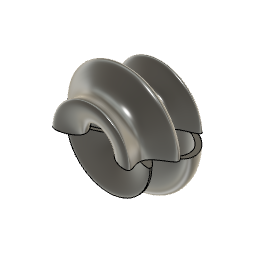
Abstract Circle v1 (Autodesk Fusion 360 design; units mm, degrees)
Autodesk Fusion 360 part; units mm, degrees
sketch "Sketch1" plane through (0, 0, 0) normal (0, 0, 1) x (1, 0, 0)
  spline S0 degree 5 poles (0, 0) (-1.4662, 0.7183) (-4.2888, 2.1966) (-8.0702, 4.4991) (-11.7581, 7.5956) (-13.3358, 11.2313) (-11.5888, 14.4429) (-6.8157, 17.1384) (-0.0929, 19.3357) (6.9956, 21.1422) (12.7502, 22.7235) (15.7261, 24.2765) (15.0691, 26.0007) (10.9795, 28.0708) (4.6166, 30.6078) (-2.3647, 33.6525) (-8.1726, 37.1355) (-11.2612, 40.8524) (-10.7466, 44.4259) (-6.6786, 47.3053) (0.2549, 48.9047) (8.9284, 48.7162) (18.0189, 46.4407) (26.218, 42.0947) (32.4803, 36.1725) (36.0989, 29.5147) (36.7231, 23.082) (34.4003, 17.7561) (29.601, 14.139) (23.273, 12.3295) (16.8297, 11.7745) (11.7686, 11.5977) (9.3075, 10.8895) (10.061, 8.9801) (13.5787, 5.7975) (18.5062, 1.8253) (23.1284, -2.1837) (25.7913, -5.4169) (25.3793, -7.2462) (21.7551, -7.4496) (15.5084, -6.1106) (9.277, -4.0415) (4.5082, -2.1134) (1.4662, -0.7183) (0, 0) knots 0 0 0 0 0 0 0.025 0.05 0.075 0.1 0.125 0.15 0.175 0.2 0.225 0.25 0.275 0.3 0.325 0.35 0.375 0.4 0.425 0.45 0.475 0.5 0.525 0.55 0.575 0.6 0.625 0.65 0.675 0.7 0.725 0.75 0.775 0.8 0.825 0.85 0.875 0.9 0.925 0.95 0.975 1 1 1 1 1 1
  spline S1 degree 5 poles (25, -5) (25.2012, -4.493) (25.9112, -3.5734) (27.8624, -2.4724) (31.8799, -1.4172) (37.7823, -0.0737) (42.9674, 2.0791) (46.1535, 5.639) (46.8953, 10.7059) (45.8562, 16.7195) (44.277, 22.7729) (43.572, 27.8507) (44.9021, 31.0817) (48.7004, 32.018) (54.3847, 30.8082) (60.8161, 27.9506) (66.6355, 24.1148) (70.6443, 19.939) (72.1699, 15.8366) (71.4326, 11.8025) (69.1917, 7.6017) (66.3861, 2.9629) (63.815, -2.2522) (61.7159, -7.8168) (59.6962, -13.1205) (57.1028, -17.417) (53.2953, -20.013) (47.9246, -20.4592) (41.2901, -18.7958) (34.3829, -15.5854) (28.4685, -11.6354) (25.5217, -8.5658) (24.7041, -6.6154) (24.7988, -5.507) (25, -5) knots 0 0 0 0 0 0 0.033333 0.066667 0.1 0.133333 0.166667 0.2 0.233333 0.266667 0.3 0.333333 0.366667 0.4 0.433333 0.466667 0.5 0.533333 0.566667 0.6 0.633333 0.666667 0.7 0.733333 0.766667 0.8 0.833333 0.866667 0.9 0.933333 0.966667 1 1 1 1 1 1
  spline S2 degree 5 poles (35, -10) (35.0607, -10.4295) (35.3776, -11.294) (36.4362, -12.596) (38.8816, -14.2347) (42.9641, -15.6792) (47.2397, -16.0554) (50.9557, -15.0177) (53.6877, -12.5043) (55.4948, -8.8331) (56.7094, -4.5257) (57.7882, -0.1787) (59.1317, 3.6928) (60.9403, 6.7779) (62.9942, 9.1614) (64.7162, 11.2631) (65.4865, 13.5525) (64.8535, 16.3559) (62.8604, 19.5601) (60.044, 22.6144) (57.1287, 24.8092) (54.8042, 25.4812) (53.4723, 24.2451) (52.9956, 21.2235) (52.8887, 16.8909) (52.5156, 11.9109) (51.2934, 6.9702) (48.87, 2.632) (45.3722, -0.8609) (41.3906, -3.5951) (37.7274, -5.8274) (35.7154, -7.4638) (35.0136, -8.7169) (34.9393, -9.5705) (35, -10) knots 0 0 0 0 0 0 0.033333 0.066667 0.1 0.133333 0.166667 0.2 0.233333 0.266667 0.3 0.333333 0.366667 0.4 0.433333 0.466667 0.5 0.533333 0.566667 0.6 0.633333 0.666667 0.7 0.733333 0.766667 0.8 0.833333 0.866667 0.9 0.933333 0.966667 1 1 1 1 1 1
  spline S3 degree 5 poles (-5, 40) (-5.2111, 40.4152) (-5.4696, 41.2213) (-5.3647, 42.3456) (-4.3046, 43.6255) (-1.8197, 44.7519) (1.3683, 45.3296) (4.8751, 45.3401) (8.4545, 44.8246) (11.9505, 43.8614) (15.2794, 42.5497) (18.399, 40.9903) (21.2854, 39.2699) (23.9015, 37.4385) (26.1878, 35.5067) (28.0807, 33.4645) (29.525, 31.2964) (30.4866, 28.9966) (30.9701, 26.5866) (31.0146, 24.1232) (30.6547, 21.6951) (29.895, 19.4209) (28.6702, 17.4504) (26.8377, 15.953) (24.2696, 15.0639) (20.933, 14.8343) (16.9651, 15.1867) (12.7774, 15.8499) (8.9528, 16.4298) (6.0946, 16.5112) (4.6846, 15.754) (4.9538, 13.9803) (6.7047, 11.2942) (9.372, 8.0446) (12.2094, 4.7046) (14.4374, 1.7775) (15.4057, -0.3074) (14.7516, -1.2965) (12.5552, -1.2109) (9.2064, -0.2562) (5.2752, 1.2664) (1.387, 3.0441) (-1.9167, 4.85) (-4.2682, 6.5957) (-5.4411, 8.274) (-5.3432, 9.9239) (-3.9995, 11.5873) (-1.5398, 13.2681) (1.8169, 14.943) (5.776, 16.5763) (9.9834, 18.1329) (14.0377, 19.5929) (17.5088, 20.963) (19.9418, 22.2952) (20.9315, 23.6722) (20.2201, 25.1795) (17.7976, 26.8812) (13.9766, 28.7973) (9.2821, 30.9121) (4.3627, 33.1784) (-0.1063, 35.5233) (-2.8344, 37.3875) (-4.203, 38.7302) (-4.7889, 39.5848) (-5, 40) knots 0 0 0 0 0 0 0.01666667 0.03333333 0.05 0.06666667 0.08333333 0.1 0.11666667 0.13333333 0.15 0.16666667 0.18333333 0.2 0.21666667 0.23333333 0.25 0.26666667 0.28333333 0.3 0.31666667 0.33333333 0.35 0.36666667 0.38333333 0.4 0.41666667 0.43333333 0.45 0.46666667 0.48333333 0.5 0.51666667 0.53333333 0.55 0.56666667 0.58333333 0.6 0.61666667 0.63333333 0.65 0.66666667 0.68333333 0.7 0.71666667 0.73333333 0.75 0.76666667 0.78333333 0.8 0.81666667 0.83333333 0.85 0.86666667 0.88333333 0.9 0.91666667 0.93333333 0.95 0.96666667 0.98333333 1 1 1 1 1 1
  line L0 (-15, 55) -> (-15, 0) construction
  point P0 (-10, 15)
  point P1 (15, 25)
  point P2 (-10, 40)
  point P3 (20, 45)
  point P4 (30, 15)
  point P5 (10, 10)
  point P6 (25, -5)
  point P7 (45, 5)
  point P8 (45, 30)
  point P9 (70, 20)
  point P10 (65, 0)
  point P11 (50, -20)
  point P12 (50, -15)
  point P13 (60, 5)
  point P14 (65, 15)
  point P15 (55, 25)
  point P16 (50, 5)
  point P17 (0, 45)
  point P18 (20, 40)
  point P19 (30, 30)
  point P20 (30, 20)
  point P21 (20, 15)
  point P22 (5, 15)
  point P23 (15, 0)
  point P24 (2.6546, 2.5063)
  point P25 (-5, 10)
  point P26 (15, 20)
  point P27 (20, 25)
  constraint coincident S0.start S0.end
  constraint coincident P6 S1.start
  constraint vertical L0
revolve "Revolve1" add sketch "Sketch1" angle 180 about axis through (-15, 55, 0) along (0, 1, 0) contours S0 S1 picked at (3.9612, 18.7116) makes body 1
sketch "Sketch2" plane through (0, 0, 0) normal (0, 0, 1) x (-1, 0, 0)
  spline S0 degree 5 poles (5, -40) (5.2111, -40.4152) (5.4696, -41.2213) (5.3647, -42.3456) (4.3046, -43.6255) (1.8197, -44.7519) (-1.3683, -45.3296) (-4.8751, -45.3401) (-8.4545, -44.8246) (-11.9505, -43.8614) (-15.2794, -42.5497) (-18.399, -40.9903) (-21.2854, -39.2699) (-23.9015, -37.4385) (-26.1878, -35.5067) (-28.0807, -33.4645) (-29.525, -31.2964) (-30.4866, -28.9966) (-30.9701, -26.5866) (-31.0146, -24.1232) (-30.6547, -21.6951) (-29.895, -19.4209) (-28.6702, -17.4504) (-26.8377, -15.953) (-24.2696, -15.0639) (-20.933, -14.8343) (-16.9651, -15.1867) (-12.7774, -15.8499) (-8.9528, -16.4298) (-6.0946, -16.5112) (-4.6846, -15.754) (-4.9538, -13.9803) (-6.7047, -11.2942) (-9.372, -8.0446) (-12.2094, -4.7046) (-14.4374, -1.7775) (-15.4057, 0.3074) (-14.7516, 1.2965) (-12.5552, 1.2109) (-9.2064, 0.2562) (-5.2752, -1.2664) (-1.387, -3.0441) (1.9167, -4.85) (4.2682, -6.5957) (5.4411, -8.274) (5.3432, -9.9239) (3.9995, -11.5873) (1.5398, -13.2681) (-1.8169, -14.943) (-5.776, -16.5763) (-9.9834, -18.1329) (-14.0377, -19.5929) (-17.5088, -20.963) (-19.9418, -22.2952) (-20.9315, -23.6722) (-20.2201, -25.1795) (-17.7976, -26.8812) (-13.9766, -28.7973) (-9.2821, -30.9121) (-4.3627, -33.1784) (0.1063, -35.5233) (2.8344, -37.3875) (4.203, -38.7302) (4.7889, -39.5848) (5, -40) knots 0 0 0 0 0 0 0.01666667 0.03333333 0.05 0.06666667 0.08333333 0.1 0.11666667 0.13333333 0.15 0.16666667 0.18333333 0.2 0.21666667 0.23333333 0.25 0.26666667 0.28333333 0.3 0.31666667 0.33333333 0.35 0.36666667 0.38333333 0.4 0.41666667 0.43333333 0.45 0.46666667 0.48333333 0.5 0.51666667 0.53333333 0.55 0.56666667 0.58333333 0.6 0.61666667 0.63333333 0.65 0.66666667 0.68333333 0.7 0.71666667 0.73333333 0.75 0.76666667 0.78333333 0.8 0.81666667 0.83333333 0.85 0.86666667 0.88333333 0.9 0.91666667 0.93333333 0.95 0.96666667 0.98333333 1 1 1 1 1 1
  spline S1 degree 5 poles (-24.9331, 6.5961) (-24.8447, 6.2472) (-24.8071, 5.9126) (-24.8207, 5.593) (-24.8854, 5.2888) (-25, 5) knots 0.981011 0.981011 0.981011 0.981011 0.981011 0.981011 1 1 1 1 1 1
  spline S2 degree 5 poles (-24.9331, 6.5961) (-24.8766, 6.6522) (-24.511, 6.9563) (-23.4266, 7.303) (-20.7676, 7.2379) (-15.5084, 6.1106) (-9.277, 4.0415) (-4.5082, 2.1134) (-1.4662, 0.7183) (0, 0) (1.4662, -0.7183) (4.2888, -2.1966) (8.0702, -4.4991) (11.7581, -7.5956) (13.3358, -11.2313) (11.5888, -14.4429) (6.8157, -17.1384) (0.0929, -19.3357) (-6.9956, -21.1422) (-12.7502, -22.7235) (-15.7261, -24.2765) (-15.0691, -26.0007) (-10.9795, -28.0708) (-4.6166, -30.6078) (2.3647, -33.6525) (8.1726, -37.1355) (11.2612, -40.8524) (10.7466, -44.4259) (6.6786, -47.3053) (-0.2549, -48.9047) (-8.9284, -48.7162) (-18.0189, -46.4407) (-26.218, -42.0947) (-32.4803, -36.1725) (-36.0989, -29.5147) (-36.7231, -23.082) (-34.4003, -17.7561) (-29.601, -14.139) (-23.273, -12.3295) (-16.8297, -11.7745) (-11.7686, -11.5977) (-9.3075, -10.8895) (-10.061, -8.9801) (-13.5787, -5.7975) (-18.479, -1.8472) (-22.1529, 1.3377) (-24.0432, 3.3814) (-24.7757, 4.5075) (-25, 5) knots 0.894761 0.894761 0.894761 0.894761 0.894761 0.894761 0.9 0.925 0.95 0.975 1 1 1 1 1 1.025 1.05 1.075 1.1 1.125 1.15 1.175 1.2 1.225 1.25 1.275 1.3 1.325 1.35 1.375 1.4 1.425 1.45 1.475 1.5 1.525 1.55 1.575 1.6 1.625 1.65 1.675 1.7 1.725 1.75 1.775 1.8 1.825 1.85 1.874311 1.874311 1.874311 1.874311 1.874311 1.874311
  spline S3 degree 5 poles (-16.2292, -23.8364) (-17.4271, -23.2603) (-19.8493, -22.1258) (-23.4682, -20.4837) (-27.875, -18.4246) (-31.7981, -16.0333) (-33.4784, -13.7428) (-32.6282, -11.4384) (-29.4887, -8.9872) (-24.9344, -6.2535) (-20.1355, -3.1315) (-16.272, 0.4251) (-14.2101, 4.3694) (-14.2367, 8.5361) (-15.6573, 12.5946) (-17.1166, 16.1133) (-17.2186, 18.6686) (-14.9957, 19.9315) (-10.571, 19.7833) (-4.9472, 18.2988) (0.4784, 15.6872) (4.3286, 12.2463) (5.6433, 8.3127) (4.4024, 4.2113) (1.4593, 0.219) (-1.9136, -3.4575) (-4.3756, -6.7114) (-4.8805, -9.5569) (-3.1115, -12.1687) (0.5871, -14.8273) (5.4566, -17.8347) (10.5156, -21.4357) (14.7619, -25.7465) (17.3982, -30.6559) (17.9408, -35.8271) (16.189, -40.8124) (12.2326, -45.1393) (6.4429, -48.4069) (-0.5252, -50.3797) (-7.7418, -51.0776) (-14.1787, -50.6946) (-18.8751, -49.5278) (-21.1178, -47.9002) (-20.5922, -46.0922) (-17.6033, -44.2536) (-13.0701, -42.3819) (-8.2045, -40.3947) (-4.2554, -38.1823) (-2.2501, -35.6623) (-2.68, -32.8472) (-5.4898, -29.837) (-9.2825, -27.3838) (-12.6622, -25.5824) (-15.0313, -24.4125) (-16.2292, -23.8364) knots 0 0 0 0 0 0 0.02 0.04 0.06 0.08 0.1 0.12 0.14 0.16 0.18 0.2 0.22 0.24 0.26 0.28 0.3 0.32 0.34 0.36 0.38 0.4 0.42 0.44 0.46 0.48 0.5 0.52 0.54 0.56 0.58 0.6 0.62 0.64 0.66 0.68 0.7 0.72 0.74 0.76 0.78 0.8 0.82 0.84 0.86 0.88 0.9 0.92 0.94 0.96 0.98 1 1 1 1 1 1
  spline S4 degree 5 poles (-25.7694, -12.1674) (-25.7825, -11.7729) (-25.6671, -10.9773) (-25.0749, -9.7601) (-23.5159, -8.0735) (-20.6215, -5.8329) (-17.2204, -3.4508) (-13.7896, -0.9382) (-10.7793, 1.6692) (-8.5529, 4.3091) (-7.3138, 6.8859) (-7.0759, 9.2792) (-7.6829, 11.3736) (-8.8213, 13.0821) (-10.0245, 14.3745) (-10.7074, 15.2956) (-10.3978, 15.9039) (-9.0379, 16.1945) (-6.963, 16.1008) (-4.6421, 15.556) (-2.4447, 14.5474) (-0.5639, 13.1308) (0.8939, 11.4021) (1.8718, 9.4817) (2.2951, 7.4933) (2.0449, 5.5462) (1.0446, 3.7184) (-0.6815, 2.0425) (-2.9154, 0.4839) (-5.2554, -1.0533) (-7.2332, -2.6925) (-8.4067, -4.5565) (-8.4548, -6.7391) (-7.2913, -9.2716) (-5.0458, -12.1269) (-1.9943, -15.2367) (1.4932, -18.5051) (5.0113, -21.8238) (8.1769, -25.0861) (10.6831, -28.2009) (12.3656, -31.1095) (13.2269, -33.7919) (13.3652, -36.2513) (12.9213, -38.5022) (12.0226, -40.5579) (10.7179, -42.4164) (8.9503, -44.0536) (6.632, -45.4361) (3.6987, -46.5296) (0.1706, -47.3093) (-3.7839, -47.7703) (-7.8021, -47.9355) (-11.4259, -47.8425) (-14.1841, -47.5337) (-15.6857, -47.0444) (-15.6982, -46.3926) (-14.2571, -45.5651) (-11.6591, -44.5209) (-8.3605, -43.211) (-4.902, -41.5931) (-1.8256, -39.6473) (0.412, -37.3949) (1.5027, -34.9059) (1.2769, -32.2767) (-0.2914, -29.6125) (-3.0887, -27.0093) (-6.8549, -24.5326) (-11.2046, -22.2095) (-15.684, -20.0386) (-19.8175, -17.9953) (-23.1595, -16.0391) (-24.9064, -14.5036) (-25.5885, -13.3446) (-25.7563, -12.562) (-25.7694, -12.1674) knots 0 0 0 0 0 0 0.01428571 0.02857143 0.04285714 0.05714286 0.07142857 0.08571429 0.1 0.11428571 0.12857143 0.14285714 0.15714286 0.17142857 0.18571429 0.2 0.21428571 0.22857143 0.24285714 0.25714286 0.27142857 0.28571429 0.3 0.31428571 0.32857143 0.34285714 0.35714286 0.37142857 0.38571429 0.4 0.41428571 0.42857143 0.44285714 0.45714286 0.47142857 0.48571429 0.5 0.51428571 0.52857143 0.54285714 0.55714286 0.57142857 0.58571429 0.6 0.61428571 0.62857143 0.64285714 0.65714286 0.67142857 0.68571429 0.7 0.71428571 0.72857143 0.74285714 0.75714286 0.77142857 0.78571429 0.8 0.81428571 0.82857143 0.84285714 0.85714286 0.87142857 0.88571429 0.9 0.91428571 0.92857143 0.94285714 0.95714286 0.97142857 0.98571429 1 1 1 1 1 1
  line L0 (20, 25) -> (20, -65) construction
  point P0 (-32.2846, -11.6951)
  point P1 (-14.5078, 5.5683)
  point P2 (-16.28, 18.8031)
  point P3 (4.5277, 10.6156)
  point P4 (-4.2061, -7.4145)
  point P5 (12.6109, -23.8034)
  point P6 (6.4559, -47.957)
  point P7 (-20.4782, -46.8275)
  point P8 (-3.8322, -37.255)
  point P9 (-9.652, 3.1385)
  point P10 (-8.7513, 12.8638)
  point P11 (-10.4409, 15.5274)
  point P12 (-5.8981, 15.796)
  point P13 (1.5468, 9.938)
  point P14 (0.0649, 2.8577)
  point P15 (-8.2477, -5.197)
  point P16 (9.7742, -27.1822)
  point P17 (12.2277, -39.921)
  point P18 (0.5402, -47.1474)
  point P19 (-15.5055, -46.7287)
  point P20 (-2.7709, -40.1256)
  point P21 (-1.9919, -28.1693)
  constraint coincident S2 P19
  constraint vertical L0
revolve "Revolve2" add sketch "Sketch2" angle 180 about axis through (-20, -25, 0) along (0, -1, 0) separate body contours S0 S2 S3 S4 | S0 S3 S4 | S0 S2 S3 S4 | S2 S3 S4 | S2 S3 S4 | S0 S2 S3 S4 | S0 S3 S4 | S0 S2 S3 S4 | S2 S3 S4 | S0 S2 S3 S4 | S0 S2 S3 S4 | S0 S2 S3 S4 | S2 S3 S4 | S0 S3 S4 makes body 2
